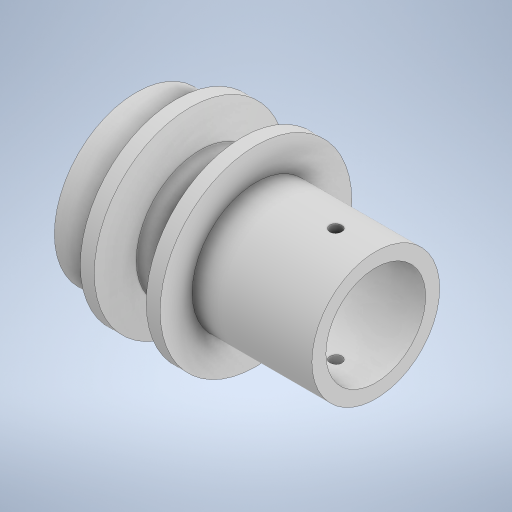
# Autodesk Inventor part: Шкив 20
Saved by Autodesk Inventor 2023 (Build 270158000, 158)
## iProperties
Created: 2022-05-01
Part Number: Шкив 20
Material: Типовые
Document SubType Name: Modeling
Designer: User
Density: 1 g/cm^3
Appearance: По умолчанию
Author: User
Autodesk Inventor part; units mm, degrees
ref_plane "YZ Plane" through (0, 0, 0) normal (1, 0, 0) x (0, 1, 0)
ref_plane "XZ Plane" through (0, 0, 0) normal (0, 1, 0) x (-1, 0, 0)
ref_plane "XY Plane" through (0, 0, 0) normal (0, 0, 1) x (1, 0, 0)
sketch "Эскиз1" plane through (0, 0, 0) normal (0, 1, 0) x (-1, 0, 0)
  line L0 (0, 24) -> (20, 24)
  line L1 (20, 24) -> (20, 0)
  line L2 (20, 0) -> (0, 0)
  line L3 (20, 24) -> (14, 24)
  line L4 (14, 24) -> (14, 16)
  line L5 (14, 16) -> (6, 16)
  line L6 (6, 16) -> (6, 24)
  line L7 (20, 0) -> (-30, 0)
  line L8 (-30, 0) -> (-30, 16)
  line L9 (-30, 16) -> (0, 16)
  line L10 (-30, 0) -> (-30, 12.5)
  line L11 (0, 16) -> (0, 24)
  line L12 (10, 16) -> (10, 24)
  line L13 (10, 24) -> (3.5, 24)
  line L14 (3.5, 24) -> (6, 16)
  line L15 (3.5, 24) -> (16.5, 24)
  line L16 (16.5, 24) -> (14, 16)
  line L17 (20, 0) -> (20, 16.5)
  line L18 (0, 0) -> (5, 0)
  line L19 (20, 16.5) -> (30, 16.5)
  line L20 (30, 16.5) -> (30, 0)
  line L21 (0, 16) -> (-5, 16)
  line L22 (-5, 0) -> (-5, 16)
  line L23 (-30, 12.5) -> (-5, 12.5)
  line L24 (30, 16.5) -> (30, 20.5)
  line L25 (30, 20.5) -> (20, 20.5)
  line L26 (-5, 12.5) -> (20, 12.5)
  point P0 (16.5, 24)
  dimension "d0" = 24
  dimension "d1" = 20
  dimension "d2" = 6
  dimension "d3" = 8
  dimension "d4" = 8
  dimension "d5" = 50
  dimension "d6" = 16
  dimension "d7" = 12.5
  dimension "d15" = 6.5
  dimension "d16" = 13
  dimension "d23" = 16.5
  dimension "d36" = 10
  dimension "d37" = 4
  constraints: 54 end point, 13 perpendicular, 12 point on line, 3 midpoint, 1 vertical
  measures "d0" distance of L2.end L0.start
  measures "d1" distance of L0.start L0.end
  measures "d2" distance of L0.end L3.end
  measures "d3" distance of L3.end L4.end
  measures "d4" distance of L4.end L5.end
  measures "d5" distance of L1.end L7.end
  measures "d6" distance of L7.end L8.end
  measures "d7" distance of L7.end L10.end
  measures "d15" distance of L12.end L13.end
  measures "d16" distance of L13.end L15.end
  measures "d23" distance of L1.end L17.end
  measures "d36" distance of L17.end L19.end
  measures "d37" distance of L19.end L24.end
sketch "Эскиз3" plane through (0, 0, 0) normal (0, 1, 0) x (-1, 0, 0)
  line L0 (0, 0) -> (-30, 0)
  line L1 (-30, 16) -> (-30, -16) projected
  line L2 (-30, 0) -> (-20, 0)
  circle A0 centre (-20, 0) radius 1.5
  dimension "d30" = 10
  dimension "d31" = 3
  constraints: 4 end point, 1 centre point, 1 coincident, 1 midpoint, 1 point on line
  measures "d30" distance of L0.end L2.end
  measures "d31" diameter of A0
revolve "Вращение4" add sketch "Эскиз1" angle 360 about axis through (-20, 0, 0) along (1, 0, 0) contours L0 L14 L5 L16 L1 L26 L22 L9 L11 | L22 L23 L8 L9 | L1 L25 L24 L19
extrude "Выдавливание4" cut sketch "Эскиз3" along normal mid plane 153
